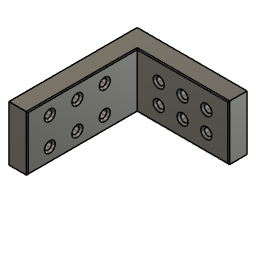
clamp v3 (Autodesk Fusion 360 design; units mm, degrees)
Autodesk Fusion 360 part; units mm, degrees
sketch "Sketch1" plane through (0, 0, 0) normal (0, 1, 0) x (1, 0, 0)
  line L0 (65, -5) -> (65, -14.5431)
  line L1 (14.2436, -31.1356) -> (24.2436, -31.1356)
  line L2 (24.2436, -101.1356) -> (14.2436, -101.1356)
  line L3 (14.2436, -101.1356) -> (14.2436, -31.1356)
  line L4 (24.2436, -31.1356) -> (74.2436, -31.1356)
  line L5 (74.2436, -31.1356) -> (74.2436, -41.1356)
  line L6 (74.2436, -41.1356) -> (24.2436, -41.1356)
  line L7 (24.2436, -41.1356) -> (24.2436, -101.1356)
  dimension "d5" = 10
  dimension "d6" = 70
  dimension "d7" = 50
  dimension "d8" = 10
  constraint vertical L0
  constraint horizontal L1
  constraint horizontal L2
  constraint vertical L3
  constraint horizontal L4
  constraint vertical L5
  constraint horizontal L6
  constraint perpendicular L2 L7
  measures "d5" distance of L1.start L1.end
  measures "d6" distance of L1.start L2.end
  measures "d7" distance of L1.end L4.end
  measures "d8" distance of L1.end L6.end
extrude "Extrude1" add sketch "Sketch1" along normal blind 30
sketch "Sketch2" plane through (0, 0, 0) normal (0, 0, 1) x (1, 0, 0)
  circle A0 centre (36, 20) radius 2
  dimension "d11" = 4
  measures "d11" diameter of A0
extrude "Extrude2" cut sketch "Sketch2" along normal blind 72
pattern_linear "R-Pattern1" count 3 spacing 13 along (1, 0, 0) count 2 spacing 11 along (0, -1, 0) of "Extrude2"
sketch "Sketch3" plane through (0, 0, 0) normal (1, 0, 0) x (0, 0, -1)
  circle A0 centre (-58.7967, 22.3764) radius 2
  dimension "d18" = 4
  measures "d18" diameter of A0
extrude "Extrude3" cut sketch "Sketch3" along normal blind 50
pattern_linear "R-Pattern2" count 3 spacing 15 along (0, 0, 1) count 2 spacing 15 along (0, -1, 0) of "Extrude3"
fillet "Fillet1" radius 0.5 6 edges at (49.2436, 30, 41.1356) (74.2436, 15, 41.1356) (24.2436, 30, 71.1356) (24.2436, 15, 101.1356) (24.2436, 0, 71.1356) (49.2436, 0, 41.1356)
chamfer "Chamfer1" distance 1 angle 45 12 edges at (34.1353, 9.7232, 41.1356) (47.1353, 9.7232, 41.1356) (60.1353, 9.7232, 41.1356) (60.1353, 20.7232, 41.1356) (47.1353, 20.7232, 41.1356) (34.1353, 20.7232, 41.1356) (24.2436, 8.0997, 60.6613) (24.2436, 8.0997, 75.6613) (24.2436, 8.0997, 90.6613) (24.2436, 23.0997, 75.6613) (24.2436, 23.0997, 90.6613) (24.2436, 23.0997, 60.6613)
